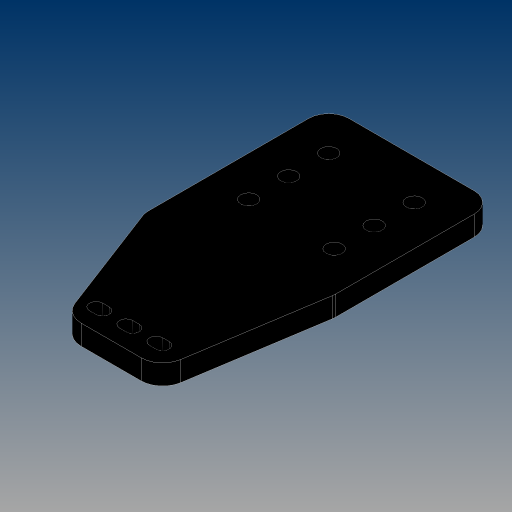
# Autodesk Inventor part: ELEV_025_CHAINCLAMP1
Saved by Autodesk Inventor 2024.3 (Build 283343000, 343)
## iProperties
Created: 2024-11-28
Part Number: ELEV_025_CHAINCLAMP1
Material: Aluminum 6061
Document SubType Name: Modeling
Designer: Kenji
Density: 2.7 g/cm^3
Appearance: Anodized - Black
Author: Kenji
Autodesk Inventor part; units mm, degrees
ref_plane "YZ Plane" through (0, 0, 0) normal (1, 0, 0) x (0, 1, 0)
ref_plane "XZ Plane" through (0, 0, 0) normal (0, 1, 0) x (-1, 0, 0)
ref_plane "XY Plane" through (0, 0, 0) normal (0, 0, 1) x (1, 0, 0)
sketch "Sketch1" plane through (0, 0, 0) normal (0, 1, 0) x (-1, 0, 0)
  line L0 (0, 25.4) -> (0, -25.4) construction
  line L1 (0, -25.4) -> (52.5018, -25.4) construction
  line L2 (15.4178, 64.3509) -> (13.335, 64.3509)
  line L3 (15.4178, 68.5165) -> (13.335, 68.5165)
  arc A0 (13.335, 68.5165) -> (13.335, 64.3509) centre (13.335, 66.4337) ccw
  arc A1 (15.4178, 64.3509) -> (15.4178, 68.5165) centre (15.4178, 66.4337) ccw
  circle A2 centre (13.335, 66.4337) radius 6.8266 construction
  line L4 (32.385, 73.2603) -> (13.335, 73.2603)
  circle A3 centre (12.7, 0) radius 2.54
  circle A4 centre (12.7, -12.7) radius 2.54
  circle A5 centre (12.7, 12.7) radius 2.54
  line L5 (12.7, -12.7) -> (12.7, 12.7) construction
  line L6 (6.5905, 67.4898) -> (0.0764, 25.8882)
  line L7 (0, 24.9059) -> (0, -19.05)
  arc A6 (0.0764, 25.8882) -> (0, 24.9059) centre (6.35, 24.9059) ccw
  line L8 (52.5018, -19.05) -> (52.5018, 31.75)
  line L9 (38.7617, 68.871) -> (52.0833, 34.0171)
  arc A7 (52.5018, 31.75) -> (52.0833, 34.0171) centre (46.1518, 31.75) ccw
  arc A8 (13.335, 73.2603) -> (6.5905, 67.4898) centre (13.335, 66.4337) ccw
  line L10 (46.1518, -25.4) -> (6.35, -25.4)
  circle A9 centre (39.8018, 12.7) radius 2.54
  circle A10 centre (39.8018, 0) radius 2.54
  circle A11 centre (39.8018, -12.7) radius 2.54
  line L11 (39.8018, -12.7) -> (39.8018, 12.7) construction
  arc A12 (46.1518, -25.4) -> (52.5018, -19.05) centre (46.1518, -19.05) ccw
  arc A13 (0, -19.05) -> (6.35, -25.4) centre (6.35, -19.05) ccw
  arc A14 (24.9428, 64.3509) -> (24.9428, 68.5165) centre (24.9428, 66.4337) ccw
  line L12 (24.9428, 64.3509) -> (22.86, 64.3509)
  line L13 (24.9428, 68.5165) -> (22.86, 68.5165)
  arc A15 (22.86, 68.5165) -> (22.86, 64.3509) centre (22.86, 66.4337) ccw
  circle A16 centre (22.86, 66.4337) radius 6.8266 construction
  arc A17 (34.4678, 64.3509) -> (34.4678, 68.5165) centre (34.4678, 66.4337) ccw
  line L14 (34.4678, 64.3509) -> (32.385, 64.3509)
  line L15 (34.4678, 68.5165) -> (32.385, 68.5165)
  arc A18 (32.385, 68.5165) -> (32.385, 64.3509) centre (32.385, 66.4337) ccw
  circle A19 centre (32.385, 66.4337) radius 6.8266 construction
  arc A20 (38.7617, 68.871) -> (32.385, 73.2603) centre (32.385, 66.4337) ccw
  line L16 (34.4678, 66.4337) -> (13.335, 66.4337) construction
  point P0 (0, 0)
  point P1 (0, 0)
  point P2 (22.86, 73.2603)
  point P3 (16.1155, 67.4898)
  point P4 (25.6405, 67.4898)
  dimension "d2" = 50.8
  dimension "d3" = 12.7
  dimension "d6" = 91.8337
  dimension "d8" = 13.335
  dimension "d9" = 2.0828
  dimension "d10" = 2.0828
  dimension "d11" = 2.0828
  dimension "d21" = 13.6533
  dimension "d31" = 5.08
  dimension "d32" = 12.7
  dimension "d33" = 12.7
  dimension "d41" = 6.35
  dimension "d42" = 6.35
  dimension "d43" = 13.335
  dimension "d45" = 12.7
  dimension "d46" = 12.7
  dimension "d47" = 6.35
  dimension "d85" = 9.525
  dimension "d90" = 27.1018
  constraints: 34 end point, 32 point on circle, 21 centre point, 14 tangent, 8 equal radius, 6 point on line, 4 coincident, 4 horizontal alignment, 4 midpoint, 4 parallel, 4 vertical, 3 horizontal, 2 collinear, 28 other
  measures "d2" distance of L0.start L0.end
  measures "d3" distance from line of L0 point (12.7, 0)
  measures "d6" distance from line of L1 A0.centre
  measures "d8" distance from line of L0 A0.centre
  measures "d9" radius of A1
  measures "d10" radius of A0
  measures "d11" distance of L2.start L2.end
  measures "d21" diameter of A2
  measures "d31" diameter of A3
  measures "d32" distance of L5.end A3.centre
  measures "d33" distance of L5.start A3.centre
  measures "d41" radius of A6
  measures "d42" radius of A7
  measures "d43" distance from line of L0 A2.centre
  measures "d45" distance of L11.start A10.centre
  measures "d46" distance from line of L8 L11.end
  measures "d47" radius of A12
  measures "d85" distance of A1.centre A14.centre
  measures "d90" distance of L5.end L11.end
extrude "Extrusion3" add sketch "Sketch1" along normal blind 6.35
body "Solid2"
